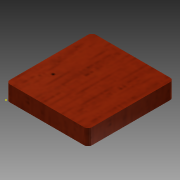
# Autodesk Inventor part: wall-front
Saved by Autodesk Inventor 2015 (Build 190159000, 159)
## iProperties
Created: 2014-07-15
Part Number: wall-front
Material: Wood (Oak)
Document SubType Name: Modeling
Designer: pc
Density: 0.76 g/cm^3
Appearance: White Oak - Natural Medium Gloss
Author: pc
Autodesk Inventor part; units mm, degrees
ref_plane "YZ Plane" through (0, 0, 0) normal (1, 0, 0) x (0, 1, 0)
ref_plane "XZ Plane" through (0, 0, 0) normal (0, 1, 0) x (-1, 0, 0)
ref_plane "XY Plane" through (0, 0, 0) normal (0, 0, 1) x (1, 0, 0)
sketch "Sketch1" plane through (0, 0, 0) normal (0, 0, 1) x (1, 0, 0)
  line L0 (0, 0) -> (42, 0)
  line L1 (42, 0) -> (42, 44)
  line L2 (42, 44) -> (0, 44)
  line L3 (0, 44) -> (0, 0)
  dimension "d0" = 42
  dimension "d1" = 44
  constraints: 8 end point, 2 parallel, 1 horizontal, 1 perpendicular
  measures "d0" distance of L2.end L1.end
  measures "d1" distance of L2.end L0.start
extrude "Extrusion1" add sketch "Sketch1" along normal blind 8
fillet "Fillet1" radius 2 1 edges at (42, 0, 4)
fillet "Fillet2" radius 2 1 edges at (42, 44, 4)
fillet "Fillet3" radius 2 1 edges at (0, 0, 4)
fillet "Fillet4" radius 2 1 edges at (0, 44, 4)
sketch "Sketch2" plane through (0, 0, 0) normal (0, 0, 1) x (1, 0, 0)
  point P0 (0, 0)
equation "\"d0\" = wallw"
equation "\"d1\" = wallh"
equation "\"d4\" = cornerrad"
equation "\"d5\" = cornerrad"
equation "\"d6\" = cornerrad"
equation "\"d7\" = cornerrad"
equation "\"printer3dtolerance\" = 0.12"
equation "\"wallw\" = 42"
equation "\"wallh\" = 44"
equation "\"cornerrad\" = 2"
equation "\"baseextra\" = 2"
equation "\"wall1_thick\" = 8"
equation "\"wall2_thick\" = 6.4"
equation "\"wall3_thick\" = 4"
equation "\"wall1slot\" = 8.12"
equation "\"wall2slot\" = 6.52"
equation "\"wall3slot\" = 4.12"
equation "\"gap2\" = 28"
equation "\"baseh\" = 79.12"
equation "\"basew\" = 44"
equation "\"base_thick\" = 6"
equation "\"base_slots_depth\" = 4"
equation "\"servosmallcircledia\" = 5.92"
equation "\"servomounth\" = 4"
equation "\"servobigcircledia\" = 11.62"
equation "\"servomountsquare\" = 6"
equation "\"distancefrombottom\" = 34"
equation "\"servopolygonr\" = 6.12"
equation "\"distancefromleft\" = 26"
equation "\"servo9gw\" = 22.8"
equation "\"servopolygonl\" = 5.92"
equation "\"wall3slotd\" = 2"
equation "\"adapterw\" = 32"
equation "\"wall3slotd_1\" = 2"
equation "\"wall3slotw\" = 36"
equation "\"adapterh\" = 16"
equation "\"armslotd\" = 2"
equation "\"armthick\" = 3"
equation "\"armw\" = 36"
body "Solid1"
